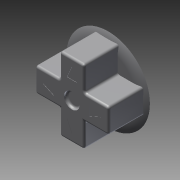
# Autodesk Inventor part: D-Pad
Saved by Autodesk Inventor 2012 SP1 (Build 160190100, 190)
## iProperties
Created: 2011-12-07
Part Number: D-Pad
Material: Default
Document SubType Name: Modeling
Designer: 133098
Density: 1 g/cm^3
Author: 133098
Autodesk Inventor part; units mm, degrees
ref_plane "YZ Plane" through (0, 0, 0) normal (1, 0, 0) x (0, 1, 0)
ref_plane "XZ Plane" through (0, 0, 0) normal (0, 1, 0) x (-1, 0, 0)
ref_plane "XY Plane" through (0, 0, 0) normal (0, 0, 1) x (1, 0, 0)
sketch "Sketch1" plane through (0, 0, 0) normal (0, 0, 1) x (1, 0, 0)
  line L0 (-8.382, 0) -> (-8.382, 2.794)
  line L1 (-8.382, 2.794) -> (-2.794, 2.794)
  line L2 (-2.794, 2.794) -> (-2.794, 8.382)
  line L3 (-2.794, 8.382) -> (0, 8.382)
  line L4 (8.382, 0) -> (8.382, 2.794)
  line L5 (8.382, 2.794) -> (2.794, 2.794)
  line L6 (2.794, 2.794) -> (2.794, 8.382)
  line L7 (2.794, 8.382) -> (0, 8.382)
  line L8 (-8.382, 0) -> (-8.382, -2.794)
  line L9 (-8.382, -2.794) -> (-2.794, -2.794)
  line L10 (-2.794, -2.794) -> (-2.794, -8.382)
  line L11 (-2.794, -8.382) -> (0, -8.382)
  line L12 (2.794, -8.382) -> (0, -8.382)
  line L13 (2.794, -2.794) -> (2.794, -8.382)
  line L14 (8.382, -2.794) -> (2.794, -2.794)
  line L15 (8.382, 0) -> (8.382, -2.794)
  point P0 (0, 0)
  dimension "d1" = 2.794
  dimension "d2" = 5.588
  constraints: 32 end point, 1 parallel
  measures "d1" distance of L0.start L0.end
  measures "d2" distance of L0.end L1.end
extrude "Extrusion1" add sketch "Sketch1" along normal blind 7.62
sketch "Sketch2" plane through (0, 0, 7.62) normal (0, 0, 1) x (1, 0, 0)
  circle A0 centre (0, 0) radius 1.778
  dimension "d7" = 3.556
  constraints: 1 centre point, 1 coincident
  measures "d7" diameter of A0
extrude "Extrusion2" cut sketch "Sketch2" against normal blind 0.635
fillet "Fillet1" radius 0.508 1 edges at (-1.778, 0, 6.985)
fillet "Fillet2" radius 0.508 16 edges at (2.794, 2.794, 3.81) (2.794, 8.382, 3.81) (2.794, 5.588, 7.62) (0, 8.382, 7.62) (-2.794, 5.588, 7.62) (-2.794, 8.382, 3.81) (-2.794, 2.794, 3.81) (-5.588, 2.794, 7.62) (-8.382, 0, 7.62) (-5.588, -2.794, 7.62) (-2.794, -5.588, 7.62) (0, -8.382, 7.62) (2.794, -5.588, 7.62) (5.588, -2.794, 7.62) (8.382, 0, 7.62) (5.588, 2.794, 7.62)
fillet "Fillet3" radius 0.508 16 edges at (-8.2332, 2.6452, 7.4712) (-8.382, 2.794, 3.556) (-8.2332, -2.6452, 7.4712) (-8.382, -2.794, 3.556) (-2.6452, -2.6452, 7.4712) (-2.794, -2.794, 3.556) (-2.6452, -8.2332, 7.4712) (-2.794, -8.382, 3.556) (2.6452, -8.2332, 7.4712) (2.794, -8.382, 3.556) (2.6452, -2.6452, 7.4712) (2.794, -2.794, 3.556) (8.2332, -2.6452, 7.4712) (8.382, -2.794, 3.556) (8.2332, 2.6452, 7.4712) (8.382, 2.794, 3.556)
sketch "Sketch3" plane through (0, 0, 7.62) normal (0, 0, 1) x (1, 0, 0)
  circle A0 centre (0, 0) radius 1.778 projected
  line L0 (3.302, 2.286) -> (7.874, 2.286) projected
  line L1 (0, 0) -> (0, 6.604)
  line L2 (0, 0) -> (6.604, 0)
  line L3 (0, 6.604) -> (0, 4.064)
  line L4 (0, 4.064) -> (-1.143, 4.064)
  line L5 (-1.143, 4.064) -> (0, 6.604)
  line L6 (0, 4.064) -> (1.143, 4.064)
  line L7 (1.143, 4.064) -> (0, 6.604)
  line L8 (6.604, 0) -> (4.064, 0)
  line L9 (4.064, 0) -> (4.064, 1.143)
  line L10 (4.064, 1.143) -> (6.604, 0)
  line L11 (4.064, 0) -> (4.064, -1.143)
  line L12 (4.064, -1.143) -> (6.604, 0)
  line L13 (0, 0) -> (0, -6.604)
  line L14 (0, -6.604) -> (0, -4.064)
  line L15 (0, -4.064) -> (-1.143, -4.064)
  line L16 (-1.143, -4.064) -> (0, -6.604)
  line L17 (0, -4.064) -> (1.143, -4.064)
  line L18 (1.143, -4.064) -> (0, -6.604)
  line L19 (0, 0) -> (-6.604, 0)
  line L20 (-6.604, 0) -> (-4.064, 0)
  line L21 (-4.064, 1.143) -> (-6.604, 0)
  line L22 (-4.064, -1.143) -> (-6.604, 0)
  line L23 (-4.064, -1.143) -> (-4.064, 1.143)
  dimension "d13" = 6.604
  dimension "d14" = 6.604
  dimension "d15" = 2.54
  dimension "d16" = 1.143
  dimension "d17" = 1.143
  dimension "d18" = 2.54
  dimension "d19" = 1.143
  dimension "d20" = 1.143
  constraints: 46 end point, 8 symmetric about line, 5 perpendicular, 4 point on line, 2 collinear
  measures "d13" distance of L1.start L1.end
  measures "d14" distance of L1.start L2.end
  measures "d15" distance of L1.end L3.end
  measures "d16" distance of L3.end L4.end
  measures "d17" distance of L3.end L6.end
  measures "d18" distance of L2.end L8.end
  measures "d19" distance of L8.end L9.end
  measures "d20" distance of L8.end L11.end
extrude "Extrusion3" cut sketch "Sketch3" against normal blind 0.0635 contours L4 L5 L1 | L1 L7 L6 | L9 L10 L2 | L2 L12 L11 | L17 L18 L13 | L13 L16 L15 | L23 L22 L19 | L19 L21 L23
sketch "Sketch4" plane through (0, 0, 0) normal (0, 0, -1) x (-1, 0, 0)
  circle A0 centre (0, 0) radius 9.525
  constraints: 1 centre point, 1 coincident
extrude "Extrusion4" add sketch "Sketch4" along normal blind 0.635
fillet "Fillet4" radius 6.35 1 edges at (9.525, 0, 0)
body "Solid1"
